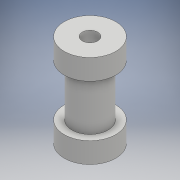
# Autodesk Inventor part: PosteLargo
Saved by Autodesk Inventor 2017 SP1 (Build 210196100, 196)
## iProperties
Part Number: PosteLargo
Material: Genérico
Document SubType Name: Modeling
Designer: Juan
Density: 1 g/cm^3
Appearance: Valor por defecto
Author: Juan
Autodesk Inventor part; units mm, degrees
ref_plane "YZ Plane" through (0, 0, 0) normal (1, 0, 0) x (0, 1, 0)
sketch "Boceto1" plane through (0, 0, 0) normal (0, 1, 0) x (-1, 0, 0)
  line L0 (0, 0) -> (5, 0)
  line L1 (5, 0) -> (5, 4)
  line L2 (5, 4) -> (3.5, 4)
  line L3 (3.5, 4) -> (3.5, 14)
  line L4 (3.5, 14) -> (5, 14)
  line L5 (5, 14) -> (5, 18)
  line L6 (5, 18) -> (0, 18)
  line L7 (0, 18) -> (0, 0)
  line L8 (0, 0) -> (0, -17) construction
  dimension "d7" = 5
  dimension "d8" = 4
  dimension "d9" = 1.5
  dimension "d10" = 10
  dimension "d11" = 4
  dimension "d12" = 5
  dimension "d13" = 18
  constraints: 18 end point, 5 perpendicular, 3 point on line, 1 coincident, 1 horizontal
  measures "d7" distance of L0.start L0.end
  measures "d8" distance of L0.end L1.end
  measures "d9" distance of L1.end L2.end
  measures "d10" distance of L2.end L3.end
  measures "d11" distance of L4.end L5.end
  measures "d12" distance of L5.end L6.end
  measures "d13" distance of L6.end L0.start
revolve "Revolución1" add sketch "Boceto1" angle 360 about axis through (0, 0, 18) along (0, 0, -1)
ref_plane "Plano de trabajo1" through (0, 0, 0) normal (0, 0, -1) x (-1, 0, 0)
sketch "Boceto2" plane through (0, 0, 0) normal (0, 0, -1) x (-1, 0, 0)
  line L0 (-5.5252, -5.4824) -> (5.4967, 5.5395) construction
  line L1 (5.4967, -5.4253) -> (-5.4966, 5.511) construction
  line L2 (5.4967, 5.5395) -> (-5.5252, -5.4824) construction
  line L3 (-5.5252, 5.5395) -> (5.4967, -5.4253) construction
  point P0 (0, 0)
  constraints: 8 end point, 2 collinear
hole "Agujero1" at (0.0143, 0, 0) direction (0, 0, 1) diameter 3 depth 5 tip angle 118
ref_plane "Plano de trabajo2" through (0, 0, 18) normal (0, 0, 1) x (1, 0, 0)
sketch "Boceto3" plane through (0, 0, 18) normal (0, 0, 1) x (1, 0, 0)
  line L0 (5.4364, 5.4796) -> (-5.5229, -5.4796) construction
  line L1 (-5.5229, 5.4796) -> (5.4075, -5.4796) construction
  point P0 (0, 0)
  constraints: 4 end point
hole "Agujero2" at (0, 0, 18) direction (0, 0, -1) diameter 3 depth 5 tip angle 118
